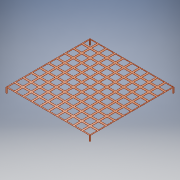
# Autodesk Inventor part: 2ft stand
Saved by Autodesk Inventor 2019 (Build 230136000, 136)
## iProperties
Created: 2020-04-28
Part Number: 2ft stand
Material: Wood (Oak)
Document SubType Name: Modeling
Designer: infinity
Density: 0.76 g/cm^3
Appearance: White Oak - Natural Medium Gloss
Author: infinity
Autodesk Inventor part; units mm, degrees
ref_plane "YZ Plane" through (0, 0, 0) normal (1, 0, 0) x (0, 1, 0)
ref_plane "XZ Plane" through (0, 0, 0) normal (0, 1, 0) x (-1, 0, 0)
ref_plane "XY Plane" through (0, 0, 0) normal (0, 0, 1) x (1, 0, 0)
sketch "Sketch1" plane through (0, 0, 0) normal (0, 1, 0) x (-1, 0, 0)
  line L0 (0, 0) -> (15240, 0)
  line L1 (15240, 0) -> (15240, -15240)
  line L2 (15240, -15240) -> (0, -15240)
  line L3 (0, -15240) -> (0, 0)
  dimension "d0" = 15240
  dimension "d1" = 15240
  constraints: 8 end point, 2 parallel, 1 horizontal, 1 perpendicular
  measures "d0" distance of L0.end L1.end
  measures "d1" distance of L0.start L0.end
extrude "Extrusion1" add sketch "Sketch1" along normal blind 25.4
sketch "Sketch2" plane through (0, 0, 0) normal (0, -1, 0) x (1, 0, 0)
  line L0 (-15240, 0) -> (0, 0) projected
  line L1 (0, 0) -> (-152.4, 0)
  line L2 (-152.4, 0) -> (-152.4, -152.4)
  line L3 (-152.4, -152.4) -> (0, -152.4)
  line L4 (0, -152.4) -> (0, 0)
  line L5 (0, 0) -> (0, -15240) projected
  line L6 (0, -15240) -> (-152.4, -15240)
  line L7 (-152.4, -15240) -> (-152.4, -15087.6)
  line L8 (-152.4, -15087.6) -> (0, -15087.6)
  line L9 (0, -15087.6) -> (0, -15240)
  line L10 (0, -15240) -> (-15240, -15240) projected
  line L11 (-15240, -15240) -> (-15087.6, -15240)
  line L12 (-15087.6, -15240) -> (-15087.6, -15087.6)
  line L13 (-15087.6, -15087.6) -> (-15240, -15087.6)
  line L14 (-15240, -15087.6) -> (-15240, -15240)
  line L15 (-15240, 0) -> (-15087.6, 0)
  line L16 (-15087.6, 0) -> (-15087.6, -152.4)
  line L17 (-15087.6, -152.4) -> (-15240, -152.4)
  line L18 (-15240, -152.4) -> (-15240, 0)
  line L19 (-152.4, -152.4) -> (-15087.6, -152.4) construction
  line L20 (-15087.6, -152.4) -> (-15087.6, -15087.6) construction
  line L21 (-15087.6, -15087.6) -> (-152.4, -15087.6) construction
  line L22 (-152.4, -15087.6) -> (-152.4, -152.4) construction
  line L23 (-15240, 0) -> (-15240, -15240) construction
  point P0 (-4572, -4572)
  dimension "d4" = 152.4
  dimension "d5" = 152.4
  dimension "d6" = 152.4
  dimension "d7" = 152.4
  constraints: 40 end point, 10 parallel, 6 point on line, 5 horizontal, 5 perpendicular
  measures "d4" distance between parallel lines of L0 L19
  measures "d5" distance from line of L0.end L2
  measures "d6" distance between parallel lines of L10 L21
  measures "d7" distance between parallel lines of L23 L20
extrude "Extrusion2" add sketch "Sketch2" along normal blind 914.4
sketch "Sketch3" plane through (0, 25.4, 0) normal (0, 1, 0) x (1, 0, 0)
  line L0 (-15080.4086, 172.1785) -> (-13861.2086, 172.1785)
  line L1 (-13861.2086, 172.1785) -> (-13861.2086, 1391.3785)
  line L2 (-13861.2086, 1391.3785) -> (-15080.4086, 1391.3785)
  line L3 (-15080.4086, 1391.3785) -> (-15080.4086, 172.1785)
  line L4 (-13556.4086, 172.1785) -> (-12337.2086, 172.1785)
  line L5 (-12337.2086, 172.1785) -> (-12337.2086, 1391.3785)
  line L6 (-12337.2086, 1391.3785) -> (-13556.4086, 1391.3785)
  line L7 (-13556.4086, 1391.3785) -> (-13556.4086, 172.1785)
  line L8 (-12032.4086, 172.1785) -> (-10813.2086, 172.1785)
  line L9 (-10813.2086, 172.1785) -> (-10813.2086, 1391.3785)
  line L10 (-10813.2086, 1391.3785) -> (-12032.4086, 1391.3785)
  line L11 (-12032.4086, 1391.3785) -> (-12032.4086, 172.1785)
  line L12 (-10508.4086, 172.1785) -> (-9289.2086, 172.1785)
  line L13 (-9289.2086, 172.1785) -> (-9289.2086, 1391.3785)
  line L14 (-9289.2086, 1391.3785) -> (-10508.4086, 1391.3785)
  line L15 (-10508.4086, 1391.3785) -> (-10508.4086, 172.1785)
  line L16 (-8984.4086, 172.1785) -> (-7765.2086, 172.1785)
  line L17 (-7765.2086, 172.1785) -> (-7765.2086, 1391.3785)
  line L18 (-7765.2086, 1391.3785) -> (-8984.4086, 1391.3785)
  line L19 (-8984.4086, 1391.3785) -> (-8984.4086, 172.1785)
  line L20 (-7460.4086, 172.1785) -> (-6241.2086, 172.1785)
  line L21 (-6241.2086, 172.1785) -> (-6241.2086, 1391.3785)
  line L22 (-6241.2086, 1391.3785) -> (-7460.4086, 1391.3785)
  line L23 (-7460.4086, 1391.3785) -> (-7460.4086, 172.1785)
  line L24 (-15080.4086, 1696.1785) -> (-13861.2086, 1696.1785)
  line L25 (-13861.2086, 1696.1785) -> (-13861.2086, 2915.3785)
  line L26 (-13861.2086, 2915.3785) -> (-15080.4086, 2915.3785)
  line L27 (-15080.4086, 2915.3785) -> (-15080.4086, 1696.1785)
  line L28 (-13556.4086, 1696.1785) -> (-12337.2086, 1696.1785)
  line L29 (-12337.2086, 1696.1785) -> (-12337.2086, 2915.3785)
  line L30 (-12337.2086, 2915.3785) -> (-13556.4086, 2915.3785)
  line L31 (-13556.4086, 2915.3785) -> (-13556.4086, 1696.1785)
  line L32 (-12032.4086, 1696.1785) -> (-10813.2086, 1696.1785)
  line L33 (-10813.2086, 1696.1785) -> (-10813.2086, 2915.3785)
  line L34 (-10813.2086, 2915.3785) -> (-12032.4086, 2915.3785)
  line L35 (-12032.4086, 2915.3785) -> (-12032.4086, 1696.1785)
  line L36 (-10508.4086, 1696.1785) -> (-9289.2086, 1696.1785)
  line L37 (-9289.2086, 1696.1785) -> (-9289.2086, 2915.3785)
  line L38 (-9289.2086, 2915.3785) -> (-10508.4086, 2915.3785)
  line L39 (-10508.4086, 2915.3785) -> (-10508.4086, 1696.1785)
  line L40 (-8984.4086, 1696.1785) -> (-7765.2086, 1696.1785)
  line L41 (-7765.2086, 1696.1785) -> (-7765.2086, 2915.3785)
  line L42 (-7765.2086, 2915.3785) -> (-8984.4086, 2915.3785)
  line L43 (-8984.4086, 2915.3785) -> (-8984.4086, 1696.1785)
  line L44 (-7460.4086, 1696.1785) -> (-6241.2086, 1696.1785)
  line L45 (-6241.2086, 1696.1785) -> (-6241.2086, 2915.3785)
  line L46 (-6241.2086, 2915.3785) -> (-7460.4086, 2915.3785)
  line L47 (-7460.4086, 2915.3785) -> (-7460.4086, 1696.1785)
  line L48 (-15080.4086, 3220.1785) -> (-13861.2086, 3220.1785)
  line L49 (-13861.2086, 3220.1785) -> (-13861.2086, 4439.3785)
  line L50 (-13861.2086, 4439.3785) -> (-15080.4086, 4439.3785)
  line L51 (-15080.4086, 4439.3785) -> (-15080.4086, 3220.1785)
  line L52 (-13556.4086, 3220.1785) -> (-12337.2086, 3220.1785)
  line L53 (-12337.2086, 3220.1785) -> (-12337.2086, 4439.3785)
  line L54 (-12337.2086, 4439.3785) -> (-13556.4086, 4439.3785)
  line L55 (-13556.4086, 4439.3785) -> (-13556.4086, 3220.1785)
  line L56 (-12032.4086, 3220.1785) -> (-10813.2086, 3220.1785)
  line L57 (-10813.2086, 3220.1785) -> (-10813.2086, 4439.3785)
  line L58 (-10813.2086, 4439.3785) -> (-12032.4086, 4439.3785)
  line L59 (-12032.4086, 4439.3785) -> (-12032.4086, 3220.1785)
  line L60 (-10508.4086, 3220.1785) -> (-9289.2086, 3220.1785)
  line L61 (-9289.2086, 3220.1785) -> (-9289.2086, 4439.3785)
  line L62 (-9289.2086, 4439.3785) -> (-10508.4086, 4439.3785)
  line L63 (-10508.4086, 4439.3785) -> (-10508.4086, 3220.1785)
  line L64 (-8984.4086, 3220.1785) -> (-7765.2086, 3220.1785)
  line L65 (-7765.2086, 3220.1785) -> (-7765.2086, 4439.3785)
  line L66 (-7765.2086, 4439.3785) -> (-8984.4086, 4439.3785)
  line L67 (-8984.4086, 4439.3785) -> (-8984.4086, 3220.1785)
  line L68 (-7460.4086, 3220.1785) -> (-6241.2086, 3220.1785)
  line L69 (-6241.2086, 3220.1785) -> (-6241.2086, 4439.3785)
  line L70 (-6241.2086, 4439.3785) -> (-7460.4086, 4439.3785)
  line L71 (-7460.4086, 4439.3785) -> (-7460.4086, 3220.1785)
  line L72 (-15080.4086, 4744.1785) -> (-13861.2086, 4744.1785)
  line L73 (-13861.2086, 4744.1785) -> (-13861.2086, 5963.3785)
  line L74 (-13861.2086, 5963.3785) -> (-15080.4086, 5963.3785)
  line L75 (-15080.4086, 5963.3785) -> (-15080.4086, 4744.1785)
  line L76 (-13556.4086, 4744.1785) -> (-12337.2086, 4744.1785)
  line L77 (-12337.2086, 4744.1785) -> (-12337.2086, 5963.3785)
  line L78 (-12337.2086, 5963.3785) -> (-13556.4086, 5963.3785)
  line L79 (-13556.4086, 5963.3785) -> (-13556.4086, 4744.1785)
  line L80 (-12032.4086, 4744.1785) -> (-10813.2086, 4744.1785)
  line L81 (-10813.2086, 4744.1785) -> (-10813.2086, 5963.3785)
  line L82 (-10813.2086, 5963.3785) -> (-12032.4086, 5963.3785)
  line L83 (-12032.4086, 5963.3785) -> (-12032.4086, 4744.1785)
  line L84 (-10508.4086, 4744.1785) -> (-9289.2086, 4744.1785)
  line L85 (-9289.2086, 4744.1785) -> (-9289.2086, 5963.3785)
  line L86 (-9289.2086, 5963.3785) -> (-10508.4086, 5963.3785)
  line L87 (-10508.4086, 5963.3785) -> (-10508.4086, 4744.1785)
  line L88 (-8984.4086, 4744.1785) -> (-7765.2086, 4744.1785)
  line L89 (-7765.2086, 4744.1785) -> (-7765.2086, 5963.3785)
  line L90 (-7765.2086, 5963.3785) -> (-8984.4086, 5963.3785)
  line L91 (-8984.4086, 5963.3785) -> (-8984.4086, 4744.1785)
  line L92 (-7460.4086, 4744.1785) -> (-6241.2086, 4744.1785)
  line L93 (-6241.2086, 4744.1785) -> (-6241.2086, 5963.3785)
  line L94 (-6241.2086, 5963.3785) -> (-7460.4086, 5963.3785)
  line L95 (-7460.4086, 5963.3785) -> (-7460.4086, 4744.1785)
  line L96 (-15080.4086, 6268.1785) -> (-13861.2086, 6268.1785)
  line L97 (-13861.2086, 6268.1785) -> (-13861.2086, 7487.3785)
  line L98 (-13861.2086, 7487.3785) -> (-15080.4086, 7487.3785)
  line L99 (-15080.4086, 7487.3785) -> (-15080.4086, 6268.1785)
  line L100 (-13556.4086, 6268.1785) -> (-12337.2086, 6268.1785)
  line L101 (-12337.2086, 6268.1785) -> (-12337.2086, 7487.3785)
  line L102 (-12337.2086, 7487.3785) -> (-13556.4086, 7487.3785)
  line L103 (-13556.4086, 7487.3785) -> (-13556.4086, 6268.1785)
  line L104 (-12032.4086, 6268.1785) -> (-10813.2086, 6268.1785)
  line L105 (-10813.2086, 6268.1785) -> (-10813.2086, 7487.3785)
  line L106 (-10813.2086, 7487.3785) -> (-12032.4086, 7487.3785)
  line L107 (-12032.4086, 7487.3785) -> (-12032.4086, 6268.1785)
  line L108 (-10508.4086, 6268.1785) -> (-9289.2086, 6268.1785)
  line L109 (-9289.2086, 6268.1785) -> (-9289.2086, 7487.3785)
  line L110 (-9289.2086, 7487.3785) -> (-10508.4086, 7487.3785)
  line L111 (-10508.4086, 7487.3785) -> (-10508.4086, 6268.1785)
  line L112 (-8984.4086, 6268.1785) -> (-7765.2086, 6268.1785)
  line L113 (-7765.2086, 6268.1785) -> (-7765.2086, 7487.3785)
  line L114 (-7765.2086, 7487.3785) -> (-8984.4086, 7487.3785)
  line L115 (-8984.4086, 7487.3785) -> (-8984.4086, 6268.1785)
  line L116 (-7460.4086, 6268.1785) -> (-6241.2086, 6268.1785)
  line L117 (-6241.2086, 6268.1785) -> (-6241.2086, 7487.3785)
  line L118 (-6241.2086, 7487.3785) -> (-7460.4086, 7487.3785)
  line L119 (-7460.4086, 7487.3785) -> (-7460.4086, 6268.1785)
  line L120 (-15080.4086, 7792.1785) -> (-13861.2086, 7792.1785)
  line L121 (-13861.2086, 7792.1785) -> (-13861.2086, 9011.3785)
  line L122 (-13861.2086, 9011.3785) -> (-15080.4086, 9011.3785)
  line L123 (-15080.4086, 9011.3785) -> (-15080.4086, 7792.1785)
  line L124 (-13556.4086, 7792.1785) -> (-12337.2086, 7792.1785)
  line L125 (-12337.2086, 7792.1785) -> (-12337.2086, 9011.3785)
  line L126 (-12337.2086, 9011.3785) -> (-13556.4086, 9011.3785)
  line L127 (-13556.4086, 9011.3785) -> (-13556.4086, 7792.1785)
  line L128 (-12032.4086, 7792.1785) -> (-10813.2086, 7792.1785)
  line L129 (-10813.2086, 7792.1785) -> (-10813.2086, 9011.3785)
  line L130 (-10813.2086, 9011.3785) -> (-12032.4086, 9011.3785)
  line L131 (-12032.4086, 9011.3785) -> (-12032.4086, 7792.1785)
  line L132 (-10508.4086, 7792.1785) -> (-9289.2086, 7792.1785)
  line L133 (-9289.2086, 7792.1785) -> (-9289.2086, 9011.3785)
  line L134 (-9289.2086, 9011.3785) -> (-10508.4086, 9011.3785)
  line L135 (-10508.4086, 9011.3785) -> (-10508.4086, 7792.1785)
  line L136 (-8984.4086, 7792.1785) -> (-7765.2086, 7792.1785)
  line L137 (-7765.2086, 7792.1785) -> (-7765.2086, 9011.3785)
  line L138 (-7765.2086, 9011.3785) -> (-8984.4086, 9011.3785)
  line L139 (-8984.4086, 9011.3785) -> (-8984.4086, 7792.1785)
  line L140 (-7460.4086, 7792.1785) -> (-6241.2086, 7792.1785)
  line L141 (-6241.2086, 7792.1785) -> (-6241.2086, 9011.3785)
  line L142 (-6241.2086, 9011.3785) -> (-7460.4086, 9011.3785)
  line L143 (-7460.4086, 9011.3785) -> (-7460.4086, 7792.1785)
  line L144 (-5936.4086, 172.1785) -> (-4717.2086, 172.1785)
  line L145 (-4717.2086, 172.1785) -> (-4717.2086, 1391.3785)
  line L146 (-4717.2086, 1391.3785) -> (-5936.4086, 1391.3785)
  line L147 (-5936.4086, 1391.3785) -> (-5936.4086, 172.1785)
  line L148 (-5936.4086, 1696.1785) -> (-4717.2086, 1696.1785)
  line L149 (-4717.2086, 1696.1785) -> (-4717.2086, 2915.3785)
  line L150 (-4717.2086, 2915.3785) -> (-5936.4086, 2915.3785)
  line L151 (-5936.4086, 2915.3785) -> (-5936.4086, 1696.1785)
  line L152 (-5936.4086, 3220.1785) -> (-4717.2086, 3220.1785)
  line L153 (-4717.2086, 3220.1785) -> (-4717.2086, 4439.3785)
  line L154 (-4717.2086, 4439.3785) -> (-5936.4086, 4439.3785)
  line L155 (-5936.4086, 4439.3785) -> (-5936.4086, 3220.1785)
  line L156 (-5936.4086, 4744.1785) -> (-4717.2086, 4744.1785)
  line L157 (-4717.2086, 4744.1785) -> (-4717.2086, 5963.3785)
  line L158 (-4717.2086, 5963.3785) -> (-5936.4086, 5963.3785)
  line L159 (-5936.4086, 5963.3785) -> (-5936.4086, 4744.1785)
  line L160 (-5936.4086, 6268.1785) -> (-4717.2086, 6268.1785)
  line L161 (-4717.2086, 6268.1785) -> (-4717.2086, 7487.3785)
  line L162 (-4717.2086, 7487.3785) -> (-5936.4086, 7487.3785)
  line L163 (-5936.4086, 7487.3785) -> (-5936.4086, 6268.1785)
  line L164 (-5936.4086, 7792.1785) -> (-4717.2086, 7792.1785)
  line L165 (-4717.2086, 7792.1785) -> (-4717.2086, 9011.3785)
  line L166 (-4717.2086, 9011.3785) -> (-5936.4086, 9011.3785)
  line L167 (-5936.4086, 9011.3785) -> (-5936.4086, 7792.1785)
  line L168 (-4412.4086, 172.1785) -> (-3193.2086, 172.1785)
  line L169 (-3193.2086, 172.1785) -> (-3193.2086, 1391.3785)
  line L170 (-3193.2086, 1391.3785) -> (-4412.4086, 1391.3785)
  line L171 (-4412.4086, 1391.3785) -> (-4412.4086, 172.1785)
  line L172 (-4412.4086, 1696.1785) -> (-3193.2086, 1696.1785)
  line L173 (-3193.2086, 1696.1785) -> (-3193.2086, 2915.3785)
  line L174 (-3193.2086, 2915.3785) -> (-4412.4086, 2915.3785)
  line L175 (-4412.4086, 2915.3785) -> (-4412.4086, 1696.1785)
  line L176 (-4412.4086, 3220.1785) -> (-3193.2086, 3220.1785)
  line L177 (-3193.2086, 3220.1785) -> (-3193.2086, 4439.3785)
  line L178 (-3193.2086, 4439.3785) -> (-4412.4086, 4439.3785)
  line L179 (-4412.4086, 4439.3785) -> (-4412.4086, 3220.1785)
  line L180 (-4412.4086, 4744.1785) -> (-3193.2086, 4744.1785)
  line L181 (-3193.2086, 4744.1785) -> (-3193.2086, 5963.3785)
  line L182 (-3193.2086, 5963.3785) -> (-4412.4086, 5963.3785)
  line L183 (-4412.4086, 5963.3785) -> (-4412.4086, 4744.1785)
  line L184 (-4412.4086, 6268.1785) -> (-3193.2086, 6268.1785)
  line L185 (-3193.2086, 6268.1785) -> (-3193.2086, 7487.3785)
  line L186 (-3193.2086, 7487.3785) -> (-4412.4086, 7487.3785)
  line L187 (-4412.4086, 7487.3785) -> (-4412.4086, 6268.1785)
  line L188 (-4412.4086, 7792.1785) -> (-3193.2086, 7792.1785)
  line L189 (-3193.2086, 7792.1785) -> (-3193.2086, 9011.3785)
  line L190 (-3193.2086, 9011.3785) -> (-4412.4086, 9011.3785)
  line L191 (-4412.4086, 9011.3785) -> (-4412.4086, 7792.1785)
  line L192 (-2888.4086, 172.1785) -> (-1669.2086, 172.1785)
  line L193 (-1669.2086, 172.1785) -> (-1669.2086, 1391.3785)
  line L194 (-1669.2086, 1391.3785) -> (-2888.4086, 1391.3785)
  line L195 (-2888.4086, 1391.3785) -> (-2888.4086, 172.1785)
  line L196 (-2888.4086, 1696.1785) -> (-1669.2086, 1696.1785)
  line L197 (-1669.2086, 1696.1785) -> (-1669.2086, 2915.3785)
  line L198 (-1669.2086, 2915.3785) -> (-2888.4086, 2915.3785)
  line L199 (-2888.4086, 2915.3785) -> (-2888.4086, 1696.1785)
  line L200 (-2888.4086, 3220.1785) -> (-1669.2086, 3220.1785)
  line L201 (-1669.2086, 3220.1785) -> (-1669.2086, 4439.3785)
  line L202 (-1669.2086, 4439.3785) -> (-2888.4086, 4439.3785)
  line L203 (-2888.4086, 4439.3785) -> (-2888.4086, 3220.1785)
  line L204 (-2888.4086, 4744.1785) -> (-1669.2086, 4744.1785)
  line L205 (-1669.2086, 4744.1785) -> (-1669.2086, 5963.3785)
  line L206 (-1669.2086, 5963.3785) -> (-2888.4086, 5963.3785)
  line L207 (-2888.4086, 5963.3785) -> (-2888.4086, 4744.1785)
  line L208 (-2888.4086, 6268.1785) -> (-1669.2086, 6268.1785)
  line L209 (-1669.2086, 6268.1785) -> (-1669.2086, 7487.3785)
  line L210 (-1669.2086, 7487.3785) -> (-2888.4086, 7487.3785)
  line L211 (-2888.4086, 7487.3785) -> (-2888.4086, 6268.1785)
  line L212 (-2888.4086, 7792.1785) -> (-1669.2086, 7792.1785)
  line L213 (-1669.2086, 7792.1785) -> (-1669.2086, 9011.3785)
  line L214 (-1669.2086, 9011.3785) -> (-2888.4086, 9011.3785)
  line L215 (-2888.4086, 9011.3785) -> (-2888.4086, 7792.1785)
  line L216 (-1364.4086, 172.1785) -> (-145.2086, 172.1785)
  line L217 (-145.2086, 172.1785) -> (-145.2086, 1391.3785)
  line L218 (-145.2086, 1391.3785) -> (-1364.4086, 1391.3785)
  line L219 (-1364.4086, 1391.3785) -> (-1364.4086, 172.1785)
  line L220 (-1364.4086, 1696.1785) -> (-145.2086, 1696.1785)
  line L221 (-145.2086, 1696.1785) -> (-145.2086, 2915.3785)
  line L222 (-145.2086, 2915.3785) -> (-1364.4086, 2915.3785)
  line L223 (-1364.4086, 2915.3785) -> (-1364.4086, 1696.1785)
  line L224 (-1364.4086, 3220.1785) -> (-145.2086, 3220.1785)
  line L225 (-145.2086, 3220.1785) -> (-145.2086, 4439.3785)
  line L226 (-145.2086, 4439.3785) -> (-1364.4086, 4439.3785)
  line L227 (-1364.4086, 4439.3785) -> (-1364.4086, 3220.1785)
  line L228 (-1364.4086, 4744.1785) -> (-145.2086, 4744.1785)
  line L229 (-145.2086, 4744.1785) -> (-145.2086, 5963.3785)
  line L230 (-145.2086, 5963.3785) -> (-1364.4086, 5963.3785)
  line L231 (-1364.4086, 5963.3785) -> (-1364.4086, 4744.1785)
  line L232 (-1364.4086, 6268.1785) -> (-145.2086, 6268.1785)
  line L233 (-145.2086, 6268.1785) -> (-145.2086, 7487.3785)
  line L234 (-145.2086, 7487.3785) -> (-1364.4086, 7487.3785)
  line L235 (-1364.4086, 7487.3785) -> (-1364.4086, 6268.1785)
  line L236 (-1364.4086, 7792.1785) -> (-145.2086, 7792.1785)
  line L237 (-145.2086, 7792.1785) -> (-145.2086, 9011.3785)
  line L238 (-145.2086, 9011.3785) -> (-1364.4086, 9011.3785)
  line L239 (-1364.4086, 9011.3785) -> (-1364.4086, 7792.1785)
  line L240 (-15080.4086, 9316.1785) -> (-13861.2086, 9316.1785)
  line L241 (-13861.2086, 9316.1785) -> (-13861.2086, 10535.3785)
  line L242 (-13861.2086, 10535.3785) -> (-15080.4086, 10535.3785)
  line L243 (-15080.4086, 10535.3785) -> (-15080.4086, 9316.1785)
  line L244 (-13556.4086, 9316.1785) -> (-12337.2086, 9316.1785)
  line L245 (-12337.2086, 9316.1785) -> (-12337.2086, 10535.3785)
  line L246 (-12337.2086, 10535.3785) -> (-13556.4086, 10535.3785)
  line L247 (-13556.4086, 10535.3785) -> (-13556.4086, 9316.1785)
  line L248 (-12032.4086, 9316.1785) -> (-10813.2086, 9316.1785)
  line L249 (-10813.2086, 9316.1785) -> (-10813.2086, 10535.3785)
  line L250 (-10813.2086, 10535.3785) -> (-12032.4086, 10535.3785)
  line L251 (-12032.4086, 10535.3785) -> (-12032.4086, 9316.1785)
  line L252 (-10508.4086, 9316.1785) -> (-9289.2086, 9316.1785)
  line L253 (-9289.2086, 9316.1785) -> (-9289.2086, 10535.3785)
  line L254 (-9289.2086, 10535.3785) -> (-10508.4086, 10535.3785)
  line L255 (-10508.4086, 10535.3785) -> (-10508.4086, 9316.1785)
  line L256 (-8984.4086, 9316.1785) -> (-7765.2086, 9316.1785)
  line L257 (-7765.2086, 9316.1785) -> (-7765.2086, 10535.3785)
  line L258 (-7765.2086, 10535.3785) -> (-8984.4086, 10535.3785)
  line L259 (-8984.4086, 10535.3785) -> (-8984.4086, 9316.1785)
  line L260 (-7460.4086, 9316.1785) -> (-6241.2086, 9316.1785)
  line L261 (-6241.2086, 9316.1785) -> (-6241.2086, 10535.3785)
  line L262 (-6241.2086, 10535.3785) -> (-7460.4086, 10535.3785)
  line L263 (-7460.4086, 10535.3785) -> (-7460.4086, 9316.1785)
  line L264 (-5936.4086, 9316.1785) -> (-4717.2086, 9316.1785)
  line L265 (-4717.2086, 9316.1785) -> (-4717.2086, 10535.3785)
  line L266 (-4717.2086, 10535.3785) -> (-5936.4086, 10535.3785)
  line L267 (-5936.4086, 10535.3785) -> (-5936.4086, 9316.1785)
  line L268 (-4412.4086, 9316.1785) -> (-3193.2086, 9316.1785)
  line L269 (-3193.2086, 9316.1785) -> (-3193.2086, 10535.3785)
  line L270 (-3193.2086, 10535.3785) -> (-4412.4086, 10535.3785)
  line L271 (-4412.4086, 10535.3785) -> (-4412.4086, 9316.1785)
  line L272 (-2888.4086, 9316.1785) -> (-1669.2086, 9316.1785)
  line L273 (-1669.2086, 9316.1785) -> (-1669.2086, 10535.3785)
  line L274 (-1669.2086, 10535.3785) -> (-2888.4086, 10535.3785)
  line L275 (-2888.4086, 10535.3785) -> (-2888.4086, 9316.1785)
  line L276 (-1364.4086, 9316.1785) -> (-145.2086, 9316.1785)
  line L277 (-145.2086, 9316.1785) -> (-145.2086, 10535.3785)
  line L278 (-145.2086, 10535.3785) -> (-1364.4086, 10535.3785)
  line L279 (-1364.4086, 10535.3785) -> (-1364.4086, 9316.1785)
  line L280 (-15080.4086, 10840.1785) -> (-13861.2086, 10840.1785)
  line L281 (-13861.2086, 10840.1785) -> (-13861.2086, 12059.3785)
  line L282 (-13861.2086, 12059.3785) -> (-15080.4086, 12059.3785)
  line L283 (-15080.4086, 12059.3785) -> (-15080.4086, 10840.1785)
  line L284 (-13556.4086, 10840.1785) -> (-12337.2086, 10840.1785)
  line L285 (-12337.2086, 10840.1785) -> (-12337.2086, 12059.3785)
  line L286 (-12337.2086, 12059.3785) -> (-13556.4086, 12059.3785)
  line L287 (-13556.4086, 12059.3785) -> (-13556.4086, 10840.1785)
  line L288 (-12032.4086, 10840.1785) -> (-10813.2086, 10840.1785)
  line L289 (-10813.2086, 10840.1785) -> (-10813.2086, 12059.3785)
  line L290 (-10813.2086, 12059.3785) -> (-12032.4086, 12059.3785)
  line L291 (-12032.4086, 12059.3785) -> (-12032.4086, 10840.1785)
  line L292 (-10508.4086, 10840.1785) -> (-9289.2086, 10840.1785)
  line L293 (-9289.2086, 10840.1785) -> (-9289.2086, 12059.3785)
  line L294 (-9289.2086, 12059.3785) -> (-10508.4086, 12059.3785)
  line L295 (-10508.4086, 12059.3785) -> (-10508.4086, 10840.1785)
  line L296 (-8984.4086, 10840.1785) -> (-7765.2086, 10840.1785)
  line L297 (-7765.2086, 10840.1785) -> (-7765.2086, 12059.3785)
  line L298 (-7765.2086, 12059.3785) -> (-8984.4086, 12059.3785)
  line L299 (-8984.4086, 12059.3785) -> (-8984.4086, 10840.1785)
  line L300 (-7460.4086, 10840.1785) -> (-6241.2086, 10840.1785)
  line L301 (-6241.2086, 10840.1785) -> (-6241.2086, 12059.3785)
  line L302 (-6241.2086, 12059.3785) -> (-7460.4086, 12059.3785)
  line L303 (-7460.4086, 12059.3785) -> (-7460.4086, 10840.1785)
  line L304 (-5936.4086, 10840.1785) -> (-4717.2086, 10840.1785)
  line L305 (-4717.2086, 10840.1785) -> (-4717.2086, 12059.3785)
  line L306 (-4717.2086, 12059.3785) -> (-5936.4086, 12059.3785)
  line L307 (-5936.4086, 12059.3785) -> (-5936.4086, 10840.1785)
  line L308 (-4412.4086, 10840.1785) -> (-3193.2086, 10840.1785)
  line L309 (-3193.2086, 10840.1785) -> (-3193.2086, 12059.3785)
  line L310 (-3193.2086, 12059.3785) -> (-4412.4086, 12059.3785)
  line L311 (-4412.4086, 12059.3785) -> (-4412.4086, 10840.1785)
  line L312 (-2888.4086, 10840.1785) -> (-1669.2086, 10840.1785)
  line L313 (-1669.2086, 10840.1785) -> (-1669.2086, 12059.3785)
  line L314 (-1669.2086, 12059.3785) -> (-2888.4086, 12059.3785)
  line L315 (-2888.4086, 12059.3785) -> (-2888.4086, 10840.1785)
  line L316 (-1364.4086, 10840.1785) -> (-145.2086, 10840.1785)
  line L317 (-145.2086, 10840.1785) -> (-145.2086, 12059.3785)
  line L318 (-145.2086, 12059.3785) -> (-1364.4086, 12059.3785)
  line L319 (-1364.4086, 12059.3785) -> (-1364.4086, 10840.1785)
  line L320 (-15080.4086, 12364.1785) -> (-13861.2086, 12364.1785)
  line L321 (-13861.2086, 12364.1785) -> (-13861.2086, 13583.3785)
  line L322 (-13861.2086, 13583.3785) -> (-15080.4086, 13583.3785)
  line L323 (-15080.4086, 13583.3785) -> (-15080.4086, 12364.1785)
  line L324 (-13556.4086, 12364.1785) -> (-12337.2086, 12364.1785)
  line L325 (-12337.2086, 12364.1785) -> (-12337.2086, 13583.3785)
  line L326 (-12337.2086, 13583.3785) -> (-13556.4086, 13583.3785)
  line L327 (-13556.4086, 13583.3785) -> (-13556.4086, 12364.1785)
  line L328 (-12032.4086, 12364.1785) -> (-10813.2086, 12364.1785)
  line L329 (-10813.2086, 12364.1785) -> (-10813.2086, 13583.3785)
  line L330 (-10813.2086, 13583.3785) -> (-12032.4086, 13583.3785)
  line L331 (-12032.4086, 13583.3785) -> (-12032.4086, 12364.1785)
  line L332 (-10508.4086, 12364.1785) -> (-9289.2086, 12364.1785)
  line L333 (-9289.2086, 12364.1785) -> (-9289.2086, 13583.3785)
  line L334 (-9289.2086, 13583.3785) -> (-10508.4086, 13583.3785)
  line L335 (-10508.4086, 13583.3785) -> (-10508.4086, 12364.1785)
  line L336 (-8984.4086, 12364.1785) -> (-7765.2086, 12364.1785)
  line L337 (-7765.2086, 12364.1785) -> (-7765.2086, 13583.3785)
  line L338 (-7765.2086, 13583.3785) -> (-8984.4086, 13583.3785)
  line L339 (-8984.4086, 13583.3785) -> (-8984.4086, 12364.1785)
  line L340 (-7460.4086, 12364.1785) -> (-6241.2086, 12364.1785)
  line L341 (-6241.2086, 12364.1785) -> (-6241.2086, 13583.3785)
  line L342 (-6241.2086, 13583.3785) -> (-7460.4086, 13583.3785)
  line L343 (-7460.4086, 13583.3785) -> (-7460.4086, 12364.1785)
  line L344 (-5936.4086, 12364.1785) -> (-4717.2086, 12364.1785)
  line L345 (-4717.2086, 12364.1785) -> (-4717.2086, 13583.3785)
  line L346 (-4717.2086, 13583.3785) -> (-5936.4086, 13583.3785)
  line L347 (-5936.4086, 13583.3785) -> (-5936.4086, 12364.1785)
  line L348 (-4412.4086, 12364.1785) -> (-3193.2086, 12364.1785)
  line L349 (-3193.2086, 12364.1785) -> (-3193.2086, 13583.3785)
  line L350 (-3193.2086, 13583.3785) -> (-4412.4086, 13583.3785)
  line L351 (-4412.4086, 13583.3785) -> (-4412.4086, 12364.1785)
  line L352 (-2888.4086, 12364.1785) -> (-1669.2086, 12364.1785)
  line L353 (-1669.2086, 12364.1785) -> (-1669.2086, 13583.3785)
  line L354 (-1669.2086, 13583.3785) -> (-2888.4086, 13583.3785)
  line L355 (-2888.4086, 13583.3785) -> (-2888.4086, 12364.1785)
  line L356 (-1364.4086, 12364.1785) -> (-145.2086, 12364.1785)
  line L357 (-145.2086, 12364.1785) -> (-145.2086, 13583.3785)
  line L358 (-145.2086, 13583.3785) -> (-1364.4086, 13583.3785)
  line L359 (-1364.4086, 13583.3785) -> (-1364.4086, 12364.1785)
  line L360 (-15080.4086, 13888.1785) -> (-13861.2086, 13888.1785)
  line L361 (-13861.2086, 13888.1785) -> (-13861.2086, 15107.3785)
  line L362 (-13861.2086, 15107.3785) -> (-15080.4086, 15107.3785)
  line L363 (-15080.4086, 15107.3785) -> (-15080.4086, 13888.1785)
  line L364 (-13556.4086, 13888.1785) -> (-12337.2086, 13888.1785)
  line L365 (-12337.2086, 13888.1785) -> (-12337.2086, 15107.3785)
  line L366 (-12337.2086, 15107.3785) -> (-13556.4086, 15107.3785)
  line L367 (-13556.4086, 15107.3785) -> (-13556.4086, 13888.1785)
  line L368 (-12032.4086, 13888.1785) -> (-10813.2086, 13888.1785)
  line L369 (-10813.2086, 13888.1785) -> (-10813.2086, 15107.3785)
  line L370 (-10813.2086, 15107.3785) -> (-12032.4086, 15107.3785)
  line L371 (-12032.4086, 15107.3785) -> (-12032.4086, 13888.1785)
  line L372 (-10508.4086, 13888.1785) -> (-9289.2086, 13888.1785)
  line L373 (-9289.2086, 13888.1785) -> (-9289.2086, 15107.3785)
  line L374 (-9289.2086, 15107.3785) -> (-10508.4086, 15107.3785)
  line L375 (-10508.4086, 15107.3785) -> (-10508.4086, 13888.1785)
  line L376 (-8984.4086, 13888.1785) -> (-7765.2086, 13888.1785)
  line L377 (-7765.2086, 13888.1785) -> (-7765.2086, 15107.3785)
  line L378 (-7765.2086, 15107.3785) -> (-8984.4086, 15107.3785)
  line L379 (-8984.4086, 15107.3785) -> (-8984.4086, 13888.1785)
  line L380 (-7460.4086, 13888.1785) -> (-6241.2086, 13888.1785)
  line L381 (-6241.2086, 13888.1785) -> (-6241.2086, 15107.3785)
  line L382 (-6241.2086, 15107.3785) -> (-7460.4086, 15107.3785)
  line L383 (-7460.4086, 15107.3785) -> (-7460.4086, 13888.1785)
  line L384 (-5936.4086, 13888.1785) -> (-4717.2086, 13888.1785)
  line L385 (-4717.2086, 13888.1785) -> (-4717.2086, 15107.3785)
  line L386 (-4717.2086, 15107.3785) -> (-5936.4086, 15107.3785)
  line L387 (-5936.4086, 15107.3785) -> (-5936.4086, 13888.1785)
  line L388 (-4412.4086, 13888.1785) -> (-3193.2086, 13888.1785)
  line L389 (-3193.2086, 13888.1785) -> (-3193.2086, 15107.3785)
  line L390 (-3193.2086, 15107.3785) -> (-4412.4086, 15107.3785)
  line L391 (-4412.4086, 15107.3785) -> (-4412.4086, 13888.1785)
  line L392 (-2888.4086, 13888.1785) -> (-1669.2086, 13888.1785)
  line L393 (-1669.2086, 13888.1785) -> (-1669.2086, 15107.3785)
  line L394 (-1669.2086, 15107.3785) -> (-2888.4086, 15107.3785)
  line L395 (-2888.4086, 15107.3785) -> (-2888.4086, 13888.1785)
  line L396 (-1364.4086, 13888.1785) -> (-145.2086, 13888.1785)
  line L397 (-145.2086, 13888.1785) -> (-145.2086, 15107.3785)
  line L398 (-145.2086, 15107.3785) -> (-1364.4086, 15107.3785)
  line L399 (-1364.4086, 15107.3785) -> (-1364.4086, 13888.1785)
  point P0 (0, 0)
  dimension "d10" = 1219.2
  dimension "d11" = 1219.2
  dimension "d14" = 1524
  dimension "d17" = 1524
  constraints: 800 end point, 2 collinear, 2 horizontal, 2 parallel, 1 perpendicular, 1 vertical, 790 other
  measures "d10" distance of L2.end L0.start
  measures "d11" distance of L0.start L0.end
  measures "d14" distance of L0.start L4.start
  measures "d17" distance of L0.start L24.start
extrude "Extrusion3" cut sketch "Sketch3" against normal up to surface (25.4 mm away)
equation "\"d1\" = d0"
equation "\"d5\" = d4"
equation "\"d6\" = d4"
equation "\"d7\" = d6"
equation "\"d11\" = d10"
body "Solid1"
